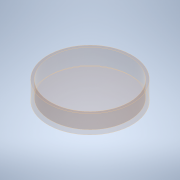
# Autodesk Inventor part: baseForBevelGearMount
Saved by Autodesk Inventor 2021 (Build 250183000, 183)
## iProperties
Created: 2020-06-18
Part Number: baseForBevelGearMount
Material: Polycarbonate, Clear
Document SubType Name: Modeling
Designer: robst
Density: 1.2 g/cm^3
Appearance: Polycarbonate - Smoked
Author: robst
Autodesk Inventor part; units mm, degrees
ref_plane "YZ Plane" through (0, 0, 0) normal (1, 0, 0) x (0, 1, 0)
ref_plane "XZ Plane" through (0, 0, 0) normal (0, 1, 0) x (-1, 0, 0)
ref_plane "XY Plane" through (0, 0, 0) normal (0, 0, 1) x (1, 0, 0)
sketch "Sketch1" plane through (0, 0, 0) normal (0, 1, 0) x (-1, 0, 0)
  circle A0 centre (0, 0) radius 101.6
  dimension "d0" = 203.2
  constraints: 1 centre point, 1 coincident
  measures "d0" diameter of A0
extrude "Extrusion1" add sketch "Sketch1" against normal blind 6.35
sketch "Sketch2" plane through (0, 0, 0) normal (0, 1, 0) x (1, 0, 0)
  circle A0 centre (0, 0) radius 101.6 projected
  circle A1 centre (0, 0) radius 101.6
  circle A2 centre (0, 0) radius 95.25
  dimension "d3" = 6.35
  constraints: 2 centre point, 2 coincident, 1 concentric
  measures "d3" radial gap between concentric circles of A2 A0
extrude "Extrusion2" add sketch "Sketch2" along normal blind 38.1
body "Solid1"
